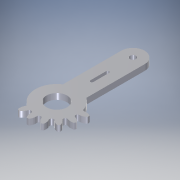
# Autodesk Inventor part: gear2
Saved by Autodesk Inventor 2016 (Build 200138000, 138)
## iProperties
Created: 2016-01-08
Part Number: gear2
Material: ABS Plastic
Document SubType Name: Modeling
Designer: Nanjar
Density: 1.06 g/cm^3
Appearance: Cool White
Author: Nanjar
Autodesk Inventor part; units mm, degrees
ref_plane "YZ Plane" through (0, 0, 0) normal (1, 0, 0) x (0, 1, 0)
ref_plane "XZ Plane" through (0, 0, 0) normal (0, 1, 0) x (-1, 0, 0)
ref_plane "XY Plane" through (0, 0, 0) normal (0, 0, 1) x (1, 0, 0)
sketch "Sketch1" plane through (0, 0, 0) normal (0, 0, 1) x (1, 0, 0)
  spline S0 degree 3 poles (-2.5287, 14.6585) (-2.4489, 14.5734) (-2.2893, 14.4032) (-2.065, 14.1344) (-1.8531, 13.8558) (-1.6566, 13.5661) (-1.4774, 13.2654) (-1.3455, 13.005) (-1.2531, 12.7907) (-1.1921, 12.6267) (-1.1387, 12.4598) (-1.1174, 12.3451) (-1.1067, 12.2878) knots 0 0 0 0 0.125009 0.250019 0.375028 0.500033 0.625034 0.750027 0.812532 0.875036 0.937535 1 1 1 1
  spline S1 degree 3 poles (-1.1067, 12.2878) (-1.1013, 12.2054) (-1.0933, 12.0819) (-1.0684, 11.9187) (-1.0411, 11.798) (-1.0079, 11.6787) (-0.9637, 11.563) (-0.9123, 11.4503) (-0.8487, 11.3439) (-0.7743, 11.2448) (-0.6883, 11.1554) (-0.5911, 11.0782) (-0.484, 11.0154) (-0.3687, 10.9696) (-0.2475, 10.9418) (-0.1236, 10.9357) (0, 10.9384) (0.1236, 10.9357) (0.2475, 10.9418) (0.3687, 10.9696) (0.484, 11.0154) (0.5911, 11.0782) (0.6883, 11.1554) (0.7743, 11.2448) (0.8487, 11.3439) (0.9123, 11.4503) (0.9637, 11.563) (1.0079, 11.6787) (1.0411, 11.798) (1.0684, 11.9187) (1.0933, 12.0819) (1.1013, 12.2054) (1.1067, 12.2878) knots 0 0 0 0 0.062498 0.093754 0.125008 0.156267 0.187517 0.21877 0.250029 0.281282 0.312529 0.343776 0.37503 0.406277 0.437515 0.468744 0.5 0.531256 0.562485 0.593723 0.62497 0.656224 0.687471 0.718718 0.749971 0.78123 0.812483 0.843733 0.874992 0.906246 0.937502 1 1 1 1
  spline S2 degree 3 poles (1.1067, 12.2878) (1.1174, 12.3451) (1.1387, 12.4598) (1.1921, 12.6267) (1.2531, 12.7907) (1.3455, 13.005) (1.4774, 13.2654) (1.6566, 13.5661) (1.8531, 13.8558) (2.065, 14.1344) (2.2893, 14.4032) (2.4489, 14.5734) (2.5287, 14.6585) knots 0 0 0 0 0.062465 0.124964 0.187468 0.249973 0.374966 0.499967 0.624972 0.749981 0.874991 1 1 1 1
  circle A0 centre (0, 0) radius 10.9375 construction
  circle A1 centre (0, 0) radius 12.3335 construction
  circle A2 centre (0, 0) radius 13.125 construction
  circle A3 centre (0, 0) radius 14.875
  point P0 (-2.2918, 14.401)
  point P1 (-2.0671, 14.1328)
  point P2 (-1.8557, 13.854)
  point P3 (-1.6594, 13.5643)
  point P4 (-1.4809, 13.2634)
  point P5 (-1.3235, 12.951)
  point P6 (-1.2545, 12.7902)
  point P7 (-1.1934, 12.6263)
  point P8 (-1.1423, 12.459)
  point P9 (-1.0859, 12.0413)
  point P10 (-1.067, 11.919)
  point P11 (-1.0402, 11.7982)
  point P12 (-1.0061, 11.6793)
  point P13 (-0.9625, 11.5635)
  point P14 (-0.9103, 11.4514)
  point P15 (-0.8469, 11.3451)
  point P16 (-0.7723, 11.2464)
  point P17 (-0.6864, 11.1574)
  point P18 (-0.5895, 11.0806)
  point P19 (-0.4826, 11.0182)
  point P20 (-0.3677, 10.9726)
  point P21 (-0.2471, 10.9455)
  point P22 (-0.1237, 10.9372)
  point P23 (0, 10.9375)
  point P24 (0.1237, 10.9372)
  point P25 (0.2471, 10.9455)
  point P26 (0.3677, 10.9726)
  point P27 (0.4826, 11.0182)
  point P28 (0.5895, 11.0806)
  point P29 (0.6864, 11.1574)
  point P30 (0.7723, 11.2464)
  point P31 (0.8469, 11.3451)
  point P32 (0.9103, 11.4514)
  point P33 (0.9625, 11.5635)
  point P34 (1.0061, 11.6793)
  point P35 (1.0402, 11.7982)
  point P36 (1.067, 11.919)
  point P37 (1.0859, 12.0413)
  point P38 (1.1423, 12.459)
  point P39 (1.1934, 12.6263)
  point P40 (1.2545, 12.7902)
  point P41 (1.3235, 12.951)
  point P42 (1.4809, 13.2634)
  point P43 (1.6594, 13.5643)
  point P44 (1.8557, 13.854)
  point P45 (2.0671, 14.1328)
  point P46 (2.2918, 14.401)
  constraints: 4 centre point, 2 point on circle, 109 other
extrude "Extrusion1" add sketch "Sketch1" against normal blind 3
extrude "Extrusion2" cut sketch "Sketch1" against normal through all contours A3 S2 S1 S0 picked at (0.2594, 13.5811)
fillet "Fillet1" radius 0.2 2 edges at (-2.5287, 14.6585, -1.5) (2.5287, 14.6585, -1.5)
pattern_circular "Circular Pattern1" count 15 over 360 about axis through (0, 0, 0) along (0, 0, -1) of "Fillet1", "Extrusion2"
sketch "Sketch9" plane through (0, 0, 0) normal (0, 1, 0) x (-1, 0, 0)
  line L0 (-6, -3) -> (6, -3)
  line L1 (6, -3) -> (6, 0)
  line L2 (6, 0) -> (-6, 0)
  line L3 (-6, 0) -> (-6, -3)
  line L4 (-6, -3) -> (6, 0) construction
  line L5 (6, -3) -> (-6, 0) construction
  line L6 (0, 0) -> (0, -1.5) construction
  point P0 (0, 0)
  dimension "d38" = 3
  dimension "d70" = 12
  constraints: 14 end point, 2 midpoint, 2 parallel, 1 coincident, 1 horizontal, 1 perpendicular
  measures "d38" distance of L1.end L0.end
  measures "d70" distance of L0.start L0.end
extrude "Extrusion8" add sketch "Sketch9" along normal blind 45
sketch "Sketch10" plane through (0, 0, 0) normal (0, 0, 1) x (1, 0, 0)
  circle A0 centre (0, 0) radius 5.25
  dimension "d41" = 10.5
  constraints: 1 centre point, 1 coincident
  measures "d41" diameter of A0
extrude "Extrusion9" cut sketch "Sketch10" against normal through all
fillet "Fillet8" radius 6 2 edges at (6, 45, -1.5) (-6, 45, -1.5)
sketch "Sketch15" plane through (0, 0, 0) normal (0, 0, 1) x (1, 0, 0)
  arc A0 (0.75, 26) -> (-0.75, 26) centre (0, 26) ccw
  arc A1 (-0.75, 18) -> (0.75, 18) centre (0, 18) ccw
  line L0 (0.75, 18) -> (0.75, 26)
  line L1 (-0.75, 18) -> (-0.75, 26)
  line L2 (0, 18) -> (0, 26) construction
  line L3 (0, 26) -> (-0.75, 26) construction
  point P0 (0, 0)
  dimension "d62" = 1.5
  dimension "d68" = 18
  dimension "d69" = 8
  constraints: 8 end point, 4 point on circle, 2 centre point, 2 vertical, 1 horizontal, 1 parallel
  measures "d62" diameter of A0
  measures "d68" distance of point (0, 0) L2.start
  measures "d69" distance of L2.start L2.end
extrude "Extrusion14" cut sketch "Sketch15" against normal through all
sketch "Sketch16" plane through (0, 0, 0) normal (0, 0, 1) x (1, 0, 0)
  arc A0 (10.402, 3.3798) -> (6, 9.1446) centre (0, 0) ccw
  line L0 (10.3806, 3.4449) -> (10.423, 3.3146) construction
  line L1 (10.402, 3.3798) -> (18.2597, 5.9329)
  line L2 (18.2597, 5.9329) -> (6, 14.4301)
  line L3 (6, 14.4301) -> (6, 9.1446)
  constraints: 8 end point, 3 point on circle, 1 centre point, 1 coincident, 1 perpendicular, 4 other
extrude "Extrusion15" cut sketch "Sketch16" against normal through all
sketch "Sketch17" plane through (0, 0, 0) normal (0, 0, 1) x (1, 0, 0)
  arc A0 (-6, 9.1446) -> (-6.4841, -8.808) centre (0, 0) ccw
  line L0 (-6.4841, -8.808) -> (-9.4042, -12.7746)
  line L1 (-15.1585, -5.0542) -> (-16.2175, -0.6874)
  line L2 (-15.1585, 5.7421) -> (-11.6769, 12.0563)
  line L3 (-6, 10.7584) -> (-6, 39) projected
  line L4 (-6, 13.433) -> (-11.6769, 12.0563)
  line L5 (-15.1585, 5.7421) -> (-16.2175, -0.6874)
  line L6 (-15.1585, -5.0542) -> (-9.4042, -12.7746)
  line L7 (-6, 13.433) -> (-6, 9.1446)
  constraints: 14 end point, 2 coincident, 2 point on circle, 1 centre point, 1 collinear, 1 perpendicular, 1 point on line, 4 other
extrude "Extrusion16" cut sketch "Sketch17" against normal through all
sketch "Sketch18" plane through (0, 0, 0) normal (0, 0, 1) x (1, 0, 0)
  arc A0 (6, 39) -> (-6, 39) centre (0, 39) ccw projected
  circle A1 centre (0, 39) radius 1.5
  point P0 (0, 0)
  dimension "d75" = 3
  constraints: 1 centre point, 1 coincident
  measures "d75" diameter of A1
extrude "Extrusion17" cut sketch "Sketch18" against normal through all
equation "\"d0\" = FaceWidth"
equation "\"Module\" = 1.75"
equation "\"PressureAngle\" = 20deg"
equation "\"UnitProfileClearance\" = 0.25"
equation "\"UnitRoundRadius\" = 0.35"
equation "\"HeadDiameter\" = 29.75"
equation "\"RootDiameter\" = 21.875"
equation "\"BaseDiameter\" = 24.66693"
equation "\"PitchDiameter\" = 26.25"
equation "\"FaceWidth\" = 3"
equation "\"HelixAngle\" = 0"
equation "\"UnitCorrection\" = 0"
equation "\"UnitAddendumModification\" = 0"
equation "\"CircularPitch\" = 5.497787"
equation "\"UnitBacklashShift\" = 0"
equation "\"TotalToolShift\" = 0"
equation "\"IsInternal\" = 0"
body "Solid1"
